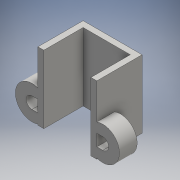
# Autodesk Inventor part: przedluzone_mocowanie
Saved by Autodesk Inventor 2016 (Build 200138000, 138)
## iProperties
Created: 2015-11-10
Part Number: przedluzone_mocowanie
Material: Ogólny
Document SubType Name: Modeling
Designer: Mrianura
Density: 1 g/cm^3
Appearance: Domyślna
Author: Mrianura
Autodesk Inventor part; units mm, degrees
ref_plane "YZ Plane" through (0, 0, 0) normal (1, 0, 0) x (0, 1, 0)
ref_plane "XZ Plane" through (0, 0, 0) normal (0, 1, 0) x (-1, 0, 0)
ref_plane "XY Plane" through (0, 0, 0) normal (0, 0, 1) x (1, 0, 0)
sketch "Szkic1" plane through (0, 0, 0) normal (0, 1, 0) x (-1, 0, 0)
  line L0 (0, 0) -> (0, 17.3)
  line L1 (0, 17.3) -> (15, 17.3)
  line L2 (15, 17.3) -> (15, 0)
  line L3 (15, 0) -> (0, 0)
  line L4 (0, 0) -> (0, 4.25)
  line L5 (0, 4.25) -> (-1.5, 4.25)
  line L6 (-1.5, 4.25) -> (16.5, 4.25)
  circle A0 centre (-1.5, 4.25) radius 4.25
  circle A1 centre (16.5, 4.25) radius 4.25
  circle A2 centre (-1.5, 4.25) radius 1.5
  circle A3 centre (16.5, 4.25) radius 1.5
  line L7 (15, 2.75) -> (16.5, 2.75)
  line L8 (16.5, 5.75) -> (15, 5.75)
  line L9 (0, 2.75) -> (-1.5, 2.75)
  line L10 (-1.5, 5.75) -> (0, 5.75)
  dimension "d0" = 17.3
  dimension "d1" = 15
  dimension "d2" = 4.25
  dimension "d3" = 1.5
  dimension "d4" = 18
  constraints: 22 end point, 10 point on line, 5 point on circle, 4 centre point, 4 coincident, 4 perpendicular, 2 tangent, 1 parallel, 1 vertical
  measures "d0" distance of L0.start L0.end
  measures "d1" distance of L0.end L1.end
  measures "d2" distance of L0.start L4.end
  measures "d3" distance of L4.end L5.end
  measures "d4" distance of L5.end L6.end
extrude "Wyciągnięcie proste1" add sketch "Szkic1" along normal blind 11.5 contours L0 L6 A0 | L0 A0 L10 A2 L9 | L0 A0 L6 | A0 L6 A1 L2 L3 L0 | A0 L0 L1 L2 A1 L6 | A1 L2 L6 | L6 L2 A1 | A1 L2 L7 A3 L8
sketch "Szkic2" plane through (0, 0, 0) normal (0, 0, -1) x (-1, 0, 0)
  line L0 (15, 0) -> (15, 11.5) projected
  line L1 (15, 0) -> (13.5, 0)
  line L2 (0, 0) -> (15, 0) projected
  line L3 (13.5, 0) -> (13.5, 10)
  line L4 (0, 11.5) -> (15, 11.5) projected
  line L5 (13.5, 10) -> (1.5, 10)
  line L6 (1.5, 10) -> (1.5, 0)
  dimension "d7" = 1.5
  dimension "d8" = 10
  dimension "d9" = 12
  constraints: 8 end point, 3 perpendicular, 2 point on line
  measures "d7" distance of L0.start L1.end
  measures "d8" distance of L1.end L3.end
  measures "d9" distance of L3.end L5.end
extrude "Wyciągnięcie proste2" cut sketch "Szkic2" against normal blind 20
sketch "Szkic3" plane through (0, 11.5, 0) normal (0, 1, 0) x (1, 0, 0)
  line L0 (0, -17.3) -> (0, -8.2265) projected
  line L1 (0, -8.8866) -> (6.1207, -8.8866)
  line L2 (6.1207, -8.8866) -> (6.1207, 0)
  line L3 (6.1207, 0) -> (0, 0)
  line L4 (0, 0) -> (0, -8.8866)
  line L5 (-15, -8.2265) -> (-15, -17.3) projected
  line L6 (-15, -8.8866) -> (-15, 0.446)
  line L7 (-15, 0.446) -> (-21.7347, 0.446)
  line L8 (-21.7347, 0.446) -> (-21.7347, -8.8866)
  line L9 (-21.7347, -8.8866) -> (-15, -8.8866)
  constraints: 16 end point, 4 perpendicular, 4 point on line, 1 collinear, 1 horizontal, 1 vertical
extrude "Wyciągnięcie proste3" cut sketch "Szkic3" against normal blind 7
